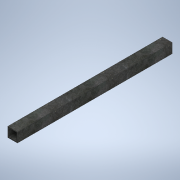
# Autodesk Inventor part: Barra_480
Saved by Autodesk Inventor 2020 (Build 240168000, 168)
## iProperties
Created: 2020-07-19
Part Number: Barra_480
Material: Acero
Document SubType Name: Modeling
Designer: louis
Density: 7.85 g/cm^3
Appearance: Placa
Author: louis
Autodesk Inventor part; units mm, degrees
ref_plane "YZ Plane" through (0, 0, 0) normal (1, 0, 0) x (0, 1, 0)
ref_plane "XZ Plane" through (0, 0, 0) normal (0, 1, 0) x (-1, 0, 0)
ref_plane "XY Plane" through (0, 0, 0) normal (0, 0, 1) x (1, 0, 0)
sketch "Boceto1" plane through (0, 0, 0) normal (0, 0, 1) x (1, 0, 0)
  line L0 (-15, 15) -> (15, 15)
  line L1 (15, 15) -> (15, -15)
  line L2 (15, -15) -> (-15, -15)
  line L3 (-15, -15) -> (-15, 15)
  line L4 (-15, 15) -> (15, -15) construction
  line L5 (15, 15) -> (-15, -15) construction
  line L6 (-12.5, 12.5) -> (12.5, 12.5)
  line L7 (12.5, 12.5) -> (12.5, -12.5)
  line L8 (12.5, -12.5) -> (-12.5, -12.5)
  line L9 (-12.5, -12.5) -> (-12.5, 12.5)
  line L10 (-12.5, 12.5) -> (12.5, -12.5) construction
  line L11 (12.5, 12.5) -> (-12.5, -12.5) construction
  point P0 (0, 0)
  dimension "d2" = 30
  dimension "d3" = 30
  dimension "d4" = 25
  dimension "d5" = 25
  constraints: 24 end point, 4 midpoint, 4 parallel, 2 horizontal, 2 perpendicular
  measures "d2" distance of L1.end L2.end
  measures "d3" distance of L0.end L1.end
  measures "d4" distance of L7.end L8.end
  measures "d5" distance of L6.end L7.end
extrude "Extrusión1" add sketch "Boceto1" against normal mid plane 480
